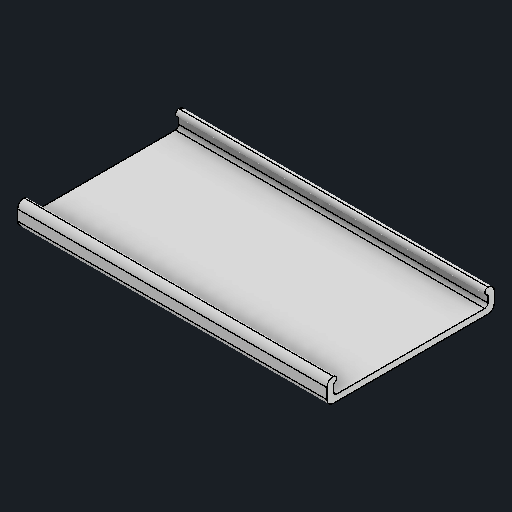
# Autodesk Inventor part: Duct Cover
Saved by Autodesk Inventor 2026.2 (Build 302298000, 298)
## iProperties
Created: 2026-06-14
Part Number: Duct Cover
Material: Generic
Document SubType Name: Modeling
Designer: JoshuaEah
Density: 1 g/cm^3
Appearance: Default
Author: JoshuaEah
Autodesk Inventor part; units mm, degrees
ref_plane "YZ Plane" through (0, 0, 0) normal (1, 0, 0) x (0, 1, 0)
ref_plane "XZ Plane" through (0, 0, 0) normal (0, 1, 0) x (-1, 0, 0)
sketch "Sketch1" plane through (0, 0, 0) normal (0, 1, 0) x (-1, 0, 0)
  line L0 (0, 0) -> (-76.2, 0)
  line L1 (-76.2, 0) -> (-76.2, -41.275)
  line L2 (-76.2, -41.275) -> (0, -41.275)
  line L3 (0, -41.275) -> (0, 0)
  line L4 (0, -39.6875) -> (-76.2, -39.6875)
  line L5 (0, -20.6375) -> (-76.2, -20.6375) construction
  dimension "d0" = 76.2
  dimension "d1" = 41.275
  dimension "d4" = 1.5875
  constraints: 12 end point, 2 midpoint, 2 parallel, 2 perpendicular, 2 point on line, 1 coincident, 1 horizontal
  measures "d0" distance of L2.end L1.end
  measures "d1" distance of L1.end L0.end
  measures "d4" distance between parallel lines of L2 L4
extrude "Extrusion1" add sketch "Sketch1" against normal blind 1.5875
ref_plane "Work Plane1" through (76.2, 0, -20.6375) normal (0, 0, -1) x (-1, 0, 0)
extrude "Extrusion2" add sketch "Sketch1" along normal blind 4.1688 contours L3 L2 L1 L4
sketch "Sketch2" plane through (0, -1.5875, 0) normal (-1, 0, 0) x (0, 0, 1)
  line L0 (-41.275, 5.7563) -> (-39.6875, 5.7563) construction
  line L1 (-39.6875, 1.5875) -> (-39.6875, 5.7563) construction
  circle A0 centre (-39.6875, 4.9625) radius 0.7937
  dimension "d7" = 1.5875
  constraints: 1 centre point, 1 point on line, 1 tangent
  measures "d7" diameter of A0
extrude "Extrusion3" add sketch "Sketch2" against normal up to surface (76.2 mm away)
fillet "Fillet1" radius 1.5875 1 edges at (38.1, 4.1688, -41.275)
mirror "Mirror1" about plane through (76.2, 0, -20.6375) normal (0, 0, -1) of "Extrusion2", "Extrusion3", "Fillet1"
fillet "Fillet2" radius 1.5875 2 edges at (38.1, -1.5875, -41.275) (38.1, -1.5875, 0)
fillet "Fillet3" radius 0.7937 2 edges at (38.1, 0, -39.6875) (38.1, 0, -1.5875)
body "Solid1"
